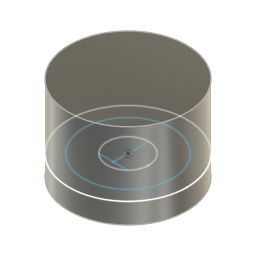
knob (Autodesk Fusion 360 design; units mm, degrees)
Autodesk Fusion 360 part; units mm, degrees
sketch "Sketch1" plane through (0, 0, 0) normal (0, 0, 1) x (1, 0, 0)
  circle A0 centre (0, 0) radius 10
  circle A1 centre (0, 0) radius 3.5
  line L0 (0, 3.5) -> (0, -2.5)
  line L1 (0, -2.5) -> (2.4495, -2.5)
  line L2 (0, -2.5) -> (-2.4495, -2.5)
  circle A2 centre (0, 0) radius 7.5
  dimension "d1" = 20
  dimension "d2" = 7
  constraint coincident A0.centre A1.centre
  constraint coincident A1 L0.start
  constraint vertical L0
  constraint coincident A1 L1.end
  constraint perpendicular L0 L1
  constraint coincident A1 L2.end
  constraint perpendicular L0 L2
  constraint concentric A0 A2
  measures "d1" diameter of A0
  measures "d2" diameter of A1
extrude "Extrude1" add sketch "Sketch1" along normal blind 12 contours A0 | A1 L0 L1 | A1 L0 L2 | A1 L1 L2 | A2
extrude "Extrude2" cut sketch "Sketch1" along normal blind 10 contours A1 L0 L1 | A1 L0 L2
sketch "Sketch2" plane through (0, 0, 0) normal (0, 0, 1) x (1, 0, 0)
extrude "Extrude3" cut 1 faces at (2.3712, -3.5556, 12) along direction (0, 0, -1) blind 1
extrude "Extrude4" add sketch "Sketch1" against normal blind 3.5 contours A0
